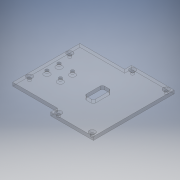
# Autodesk Inventor part: ImagineFrameTopBot
Saved by Autodesk Inventor 2018 (Build 220112000, 112)
## iProperties
Created: 2020-09-26
Part Number: ImagineFrameTopBot
Material: SAN Plastic
Document SubType Name: Modeling
Designer: Lveli
Density: 1.068 g/cm^3
Appearance: Polycarbonate - Clear
Author: Lveli
Autodesk Inventor part; units mm, degrees
ref_plane "YZ Plane" through (0, 0, 0) normal (1, 0, 0) x (0, 1, 0)
ref_plane "XZ Plane" through (0, 0, 0) normal (0, 1, 0) x (-1, 0, 0)
ref_plane "XY Plane" through (0, 0, 0) normal (0, 0, 1) x (1, 0, 0)
sketch "Sketch1" plane through (0, 0, 0) normal (0, 1, 0) x (-1, 0, 0)
  line L0 (0, 0) -> (60.325, 0)
  line L1 (60.325, 0) -> (60.325, -9.525)
  line L2 (60.325, -9.525) -> (117.475, -9.525)
  line L3 (117.475, -9.525) -> (117.475, -104.775)
  line L4 (117.475, -104.775) -> (60.325, -104.775)
  line L5 (60.325, -104.775) -> (60.325, -114.3)
  line L6 (60.325, -114.3) -> (0, -114.3)
  line L7 (0, -114.3) -> (0, 0)
  dimension "d0" = 9.525
  dimension "d1" = 95.25
  dimension "d2" = 57.15
  dimension "d3" = 60.325
  dimension "d4" = 117.475
  dimension "d5" = 114.3
  constraints: 16 end point, 6 perpendicular, 2 point on line, 1 collinear, 1 horizontal
  measures "d0" distance of L0.end L1.end
  measures "d1" distance between parallel lines of L4 L2
  measures "d2" distance of L1.end L2.end
  measures "d3" distance of L0.start L0.end
  measures "d4" distance between parallel lines of L3 L7
  measures "d5" distance between parallel lines of L6 L0
extrude "Extrusion1" add sketch "Sketch1" along normal blind 4.7625
sketch "Sketch2" plane through (0, 4.7625, 0) normal (0, 1, 0) x (1, 0, 0)
  line L0 (-117.475, 9.525) -> (-117.475, 104.775) construction
  line L1 (-117.475, 57.15) -> (0, 57.15) construction
  line L2 (-60.325, 0) -> (0, 0) construction
  line L3 (0, 0) -> (0, 114.3) construction
  line L4 (0, 114.3) -> (-60.325, 114.3) construction
  line L5 (-60.325, 114.3) -> (-60.325, 104.775) construction
  line L6 (-60.325, 104.775) -> (-117.475, 104.775) construction
  line L7 (-117.475, 104.775) -> (-117.475, 9.525) construction
  line L8 (-117.475, 9.525) -> (-60.325, 9.525) construction
  line L9 (-60.325, 9.525) -> (-60.325, 0) construction
  point P0 (-53.975, 4.7625)
  point P1 (-6.35, 4.7625)
  point P2 (-112.7125, 28.575)
  point P3 (-53.975, 109.5375)
  point P4 (-6.35, 109.5375)
  point P5 (-112.7125, 85.725)
  dimension "d8" = 6.35
  dimension "d9" = 6.35
  dimension "d10" = 4.7625
  dimension "d11" = 4.7625
  dimension "d12" = 19.05
  dimension "d13" = 4.7625
  constraints: 3 symmetric about line, 2 end point, 1 horizontal, 1 midpoint
  measures "d8" distance from line of L3 point (-6.35, 4.763)
  measures "d9" distance from line of L9 point (-53.975, 4.763)
  measures "d10" distance from line of L2 point (-53.975, 4.763)
  measures "d11" distance from line of L2 point (-6.35, 4.763)
  measures "d12" distance from line of L8 point (-112.712, 28.575)
  measures "d13" distance from line of L0 point (-112.712, 28.575)
hole "Hole1" at (-53.975, 4.7625, -4.7625) at (-6.35, 4.7625, -4.7625) at (-112.7125, 4.7625, -28.575) at (-6.35, 4.7625, -109.5375) at (-53.975, 4.7625, -109.5375) at (-112.7125, 4.7625, -85.725) direction (0, -1, 0) diameter 4.4958 end through all countersink diameter 8.4328 countersink angle 82 clearance for "Flat Head Machine Screw (82)" size "#8" standard "Ansi Unified Screw Threads"
sketch "Sketch3" plane through (0, 0, 0) normal (0, -1, 0) x (1, 0, 0)
  circle A0 centre (-53.975, -109.5375) radius 2.2479 construction
  circle A1 centre (-112.7125, -28.575) radius 2.2479 construction
  circle A2 centre (-53.975, -4.7625) radius 2.2479 construction
  circle A3 centre (-6.35, -4.7625) radius 2.2479 construction
  circle A4 centre (-6.35, -109.5375) radius 2.2479 construction
  circle A5 centre (-112.7125, -85.725) radius 2.2479 construction
  line L0 (0, 0) -> (-60.325, 0) construction
  line L1 (-60.325, 0) -> (-60.325, -9.525) construction
  line L2 (-60.325, -9.525) -> (-117.475, -9.525) construction
  line L3 (-117.475, -9.525) -> (-117.475, -104.775) construction
  line L4 (-117.475, -104.775) -> (-60.325, -104.775) construction
  line L5 (-60.325, -104.775) -> (-60.325, -114.3) construction
  line L6 (-60.325, -114.3) -> (0, -114.3) construction
  line L7 (0, -114.3) -> (0, 0) construction
  line L8 (0, -57.15) -> (-117.475, -57.15) construction
  point P0 (-88.9, -48.5775)
  point P1 (-107.95, -48.5775)
  point P2 (-88.9, -65.7225)
  point P3 (-107.95, -65.7225)
  dimension "d22" = 19.05
  dimension "d23" = 8.5725
  dimension "d24" = 8.5725
  dimension "d32" = 9.525
  constraints: 2 end point, 2 midpoint, 2 symmetric about line
  measures "d22" distance of point (-88.9, -48.578) point (-107.95, -48.577)
  measures "d23" distance from line of L8 point (-107.95, -48.577)
  measures "d24" distance from line of L8 point (-88.9, -48.578)
  measures "d32" distance from line of L3 point (-107.95, -48.577)
hole "Hole2" at (-88.9, 0, -48.5775) at (-107.95, 0, -48.5775) at (-88.9, 0, -65.7225) at (-107.95, 0, -65.7225) direction (0, 1, 0) diameter 4.4958 end through all countersink diameter 8.4328 countersink angle 82 clearance for "Flat Head Machine Screw (82)" size "#8" standard "Ansi Unified Screw Threads"
sketch "Sketch4" plane through (0, 4.7625, 0) normal (0, 1, 0) x (1, 0, 0)
  line L0 (-47.625, 44.45) -> (-53.975, 44.45)
  line L1 (-57.15, 47.625) -> (-57.15, 66.675)
  line L2 (-53.975, 69.85) -> (-47.625, 69.85)
  line L3 (-44.45, 66.675) -> (-44.45, 47.625)
  line L4 (-44.45, 44.45) -> (-57.15, 69.85) construction
  line L5 (-57.15, 44.45) -> (-44.45, 69.85) construction
  line L6 (0, 0) -> (0, 114.3) projected
  line L7 (0, 57.15) -> (-50.8, 57.15) construction
  arc A0 (-53.975, 69.85) -> (-57.15, 66.675) centre (-53.975, 66.675) ccw
  arc A1 (-44.45, 66.675) -> (-47.625, 69.85) centre (-47.625, 66.675) ccw
  arc A2 (-47.625, 44.45) -> (-44.45, 47.625) centre (-47.625, 47.625) ccw
  arc A3 (-57.15, 47.625) -> (-53.975, 44.45) centre (-53.975, 47.625) ccw
  dimension "d33" = 50.8
  dimension "d34" = 12.7
  dimension "d35" = 25.4
  dimension "d36" = 3.175
  constraints: 14 end point, 8 point on circle, 8 point on line, 8 tangent, 4 centre point, 3 equal radius, 3 midpoint, 2 horizontal, 2 parallel, 1 perpendicular
  measures "d33" distance from line of L6 L7.end
  measures "d34" distance of L4.end L5.end
  measures "d35" distance of L5.start L4.end
  measures "d36" radius of A0
extrude "Extrusion2" cut sketch "Sketch4" against normal through all
equation "\"d24\" = d23"
body "Solid1"
